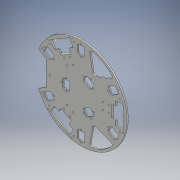
# Autodesk Inventor part: Base
Saved by Autodesk Inventor 2018 (Build 220112000, 112)
## iProperties
Created: 2017-10-12
Part Number: Base
Material: Generic
Document SubType Name: Modeling
Designer: BrisbaneMatt
Density: 1 g/cm^3
Appearance: Default
Author: BrisbaneMatt
Autodesk Inventor part; units mm, degrees
(part 1 of 2)
ref_plane "YZ Plane" through (0, 0, 0) normal (1, 0, 0) x (0, 1, 0)
ref_plane "XZ Plane" through (0, 0, 0) normal (0, 1, 0) x (-1, 0, 0)
ref_plane "XY Plane" through (0, 0, 0) normal (0, 0, 1) x (1, 0, 0)
sketch "Sketch1" plane through (0, 0, 0) normal (0, 1, 0) x (-1, 0, 0)
  circle A0 centre (0, 0) radius 105
  line L0 (0, 0) -> (105, 0) construction
  line L1 (70.1408, 71.4875) -> (26.8396, 96.4875)
  line L2 (70.1408, 71.4875) -> (61.3908, 56.332)
  line L3 (61.3908, 56.332) -> (18.0896, 81.332)
  line L4 (18.0896, 81.332) -> (26.8396, 96.4875)
  line L5 (26.8396, -96.4875) -> (70.1408, -71.4875)
  line L6 (70.1408, -71.4875) -> (61.3908, -56.332)
  line L7 (61.3908, -56.332) -> (18.0896, -81.332)
  line L8 (18.0896, -81.332) -> (26.8396, -96.4875)
  line L9 (0, 0) -> (-105, 0)
  line L10 (-96.9804, -25) -> (-96.9804, 25)
  line L11 (-96.9804, 25) -> (-79.4804, 25)
  line L12 (-79.4804, 25) -> (-79.4804, -25)
  line L13 (-79.4804, -25) -> (-96.9804, -25)
  dimension "d0" = 210
  dimension "d5" = 50
  dimension "d6" = 17.5
  dimension "d8" = 50
  dimension "d9" = 17.5
  dimension "d12" = 50
  dimension "d13" = 17.5
  constraints: 28 end point, 6 perpendicular, 3 horizontal, 1 coincident, 1 horizontal alignment, 1 vertical, 2 other
  measures "d5" distance of L1.start L1.end
  measures "d6" distance of L1.start L2.end
  measures "d8" distance of L5.start L5.end
  measures "d9" distance of L5.end L6.end
  measures "d12" distance of L10.start L10.end
  measures "d13" distance of L10.end L11.end
extrude "Extrusion1" add sketch "Sketch1" along normal blind 3
sketch "Sketch2" plane through (0, 3, 0) normal (0, 1, 0) x (1, 0, 0)
  line L0 (-61.3908, -56.332) -> (-18.0896, -81.332) projected
  line L1 (-39.7402, -68.832) -> (-24.9902, -43.2843)
  line L2 (-32.3652, -56.0582) -> (-35.7652, -61.9471)
  line L3 (-35.7652, -61.9471) -> (-42.6501, -57.9721)
  line L4 (-35.7652, -61.9471) -> (-28.9652, -50.1692)
  line L5 (-28.9652, -50.1692) -> (-35.8501, -46.1942)
  line L6 (-35.8501, -46.1942) -> (-22.0803, -54.1442)
  line L7 (-42.6501, -57.9721) -> (-28.8803, -65.9221)
  circle A0 centre (-42.6501, -57.9721) radius 1.5
  circle A1 centre (-35.8501, -46.1942) radius 1.5
  circle A2 centre (-22.0803, -54.1442) radius 1.5
  circle A3 centre (-28.8803, -65.9221) radius 1.5
  point P0 (0, 0)
  dimension "d17" = 29.5
  dimension "d18" = 6.8
  dimension "d19" = 7.95
  dimension "d20" = 13.6
  dimension "d21" = 7.95
  dimension "d22" = 15.9
  dimension "d23" = 15.9
  dimension "d24" = 3
  dimension "d25" = 3
  dimension "d26" = 3
  dimension "d27" = 3
  constraints: 14 end point, 4 centre point, 4 coincident, 4 point on line, 2 midpoint, 1 perpendicular
  measures "d17" distance of L1.start L1.end
  measures "d18" distance of L2.start L2.end
  measures "d19" distance of L2.end L3.end
  measures "d20" distance of L2.end L4.end
  measures "d21" distance of L4.end L5.end
  measures "d22" distance of L5.end L6.end
  measures "d23" distance of L3.end L7.end
  measures "d24" diameter of A0
  measures "d25" diameter of A1
  measures "d26" diameter of A2
  measures "d27" diameter of A3
extrude "Extrusion2" cut sketch "Sketch2" against normal blind 3
sketch "Sketch3" plane through (0, 3, 0) normal (0, 1, 0) x (1, 0, 0)
  line L0 (-17.4161, -70.8938) -> (-32.5784, -70.8938)
  line L1 (-32.5784, -70.8938) -> (-32.5784, -46.1015)
  line L2 (-32.5784, -46.1015) -> (-17.4161, -46.1015)
  line L3 (-17.4161, -46.1015) -> (-17.4161, -70.8938)
  line L4 (-30.5294, -62.4931) -> (-47.7406, -62.4931)
  line L5 (-47.7406, -62.4931) -> (-47.7406, -39.5448)
  line L6 (-47.7406, -39.5448) -> (-30.5294, -39.5448)
  line L7 (-30.5294, -39.5448) -> (-30.5294, -62.4931)
  point P0 (0, 0)
  constraints: 16 end point, 4 parallel, 2 horizontal, 2 perpendicular
extrude "Extrusion3" add sketch "Sketch3" against normal blind 3
sketch "Sketch4" plane through (0, 3, 0) normal (0, 1, 0) x (1, 0, 0)
  line L0 (-18.0896, -81.332) -> (-61.3908, -56.332) projected
  line L1 (-39.7402, -68.832) -> (-32.812, -72.832)
  line L2 (-32.812, -72.832) -> (-39.7402, -68.832)
  line L3 (-39.7402, -68.832) -> (-35.7402, -61.9038)
  line L4 (-35.7402, -61.9038) -> (-47.4315, -55.1538)
  line L5 (-47.4315, -55.1538) -> (-51.4315, -62.082)
  line L6 (-51.4315, -62.082) -> (-39.7402, -68.832)
  line L7 (-35.7402, -61.9038) -> (-24.0489, -68.6538)
  line L8 (-24.0489, -68.6538) -> (-28.0489, -75.582)
  line L9 (-28.0489, -75.582) -> (-32.812, -72.832)
  line L10 (-61.3908, 56.332) -> (-18.0896, 81.332) projected
  line L11 (-39.7402, 68.832) -> (-51.4315, 62.082)
  line L12 (-51.4315, 62.082) -> (-47.4315, 55.1538)
  line L13 (-47.4315, 55.1538) -> (-24.0489, 68.6538)
  line L14 (-24.0489, 68.6538) -> (-28.0489, 75.582)
  line L15 (-28.0489, 75.582) -> (-39.7402, 68.832)
  line L16 (79.4804, 25) -> (79.4804, -25) projected
  line L17 (79.4804, 0) -> (79.4804, 13.5)
  line L18 (79.4804, 13.5) -> (71.4804, 13.5)
  line L19 (71.4804, 13.5) -> (71.4804, -13.5)
  line L20 (71.4804, -13.5) -> (79.4804, -13.5)
  line L21 (79.4804, -13.5) -> (79.4804, 0)
  point P0 (0, 0)
  dimension "d32" = 8
  dimension "d33" = 8
  dimension "d34" = 13.5
  dimension "d35" = 13.5
  dimension "d36" = 13.5
  dimension "d37" = 8
  dimension "d38" = 27
  dimension "d39" = 13.5
  dimension "d40" = 8
  dimension "d41" = 27
  constraints: 38 end point, 10 perpendicular, 8 point on line, 4 collinear, 3 midpoint
  measures "d32" distance of L1.start L1.end
  measures "d33" distance of L1.start L3.end
  measures "d34" distance of L3.end L4.end
  measures "d35" distance of L3.end L7.end
  measures "d36" distance of L11.start L11.end
  measures "d37" distance of L11.end L12.end
  measures "d38" distance of L12.end L13.end
  measures "d39" distance of L17.start L17.end
  measures "d40" distance of L17.end L18.end
  measures "d41" distance of L18.end L19.end
extrude "Extrusion4" cut sketch "Sketch4" against normal blind 3
sketch "Sketch5" plane through (0, 3, 0) normal (0, 1, 0) x (1, 0, 0)
  line L0 (-47.4315, -55.1538) -> (-24.0489, -68.6538) projected
  line L1 (-35.7402, -61.9038) -> (-4.2402, -7.3442)
  line L2 (-4.2402, -7.3442) -> (-15.9315, -0.5942)
  line L3 (-15.9315, -0.5942) -> (-47.4315, -55.1538)
  line L4 (-4.2402, -7.3442) -> (7.4511, -14.0942)
  line L5 (7.4511, -14.0942) -> (-24.0489, -68.6538)
  line L6 (-24.0489, -68.6538) -> (-35.7402, -61.9038)
  line L7 (-47.4315, 55.1538) -> (-24.0489, 68.6538) projected
  line L8 (-35.7402, 61.9038) -> (-4.2402, 7.3442)
  line L9 (-4.2402, 7.3442) -> (-15.9315, 0.5942)
  line L10 (-47.4315, 55.1538) -> (-51.4315, 62.082) projected
  line L11 (-15.9315, 0.5942) -> (-47.4315, 55.1538)
  line L12 (-47.4315, 55.1538) -> (-24.0489, 68.6538)
  line L13 (-24.0489, 68.6538) -> (7.4511, 14.0942)
  line L14 (7.4511, 14.0942) -> (-4.2402, 7.3442)
  line L15 (71.4804, 13.5) -> (71.4804, -13.5) projected
  line L16 (71.4804, -13.5) -> (8.4804, -13.5)
  line L17 (71.4804, -13.5) -> (134.4804, -13.5) construction
  line L18 (79.4804, 13.5) -> (71.4804, 13.5) projected
  line L19 (71.4804, 13.5) -> (8.4804, 13.5)
  line L20 (71.4804, 13.5) -> (134.4804, 13.5) construction
  line L21 (8.4804, 13.5) -> (8.4804, -13.5)
  line L22 (-35.7402, -61.9038) -> (-47.4315, -55.1538)
  line L23 (0, 0) -> (-30, 0)
  line L24 (-30, 0) -> (-30, -10)
  line L25 (-30, -10) -> (-46, -10)
  line L26 (-46, -10) -> (-46, 10)
  line L27 (-46, 10) -> (-30, 10)
  line L28 (-30, 10) -> (-30, 0)
  line L29 (0, 0) -> (15, 25.9808)
  line L30 (15, 25.9808) -> (6.3397, 30.9808)
  line L31 (6.3397, 30.9808) -> (14.3397, 44.8372)
  line L32 (14.3397, 44.8372) -> (31.6603, 34.8372)
  line L33 (31.6603, 34.8372) -> (23.6603, 20.9808)
  line L34 (23.6603, 20.9808) -> (15, 25.9808)
  line L35 (0, 0) -> (15, -25.9808)
  line L36 (15, -25.9808) -> (6.3397, -30.9808)
  line L37 (6.3397, -30.9808) -> (14.3397, -44.8372)
  line L38 (14.3397, -44.8372) -> (31.6603, -34.8372)
  line L39 (31.6603, -34.8372) -> (23.6603, -20.9808)
  line L40 (23.6603, -20.9808) -> (15, -25.9808)
  dimension "d45" = 63
  dimension "d46" = 13.5
  dimension "d47" = 13.5
  dimension "d49" = 63
  dimension "d50" = 13.5
  dimension "d51" = 63
  dimension "d52" = 180
  dimension "d53" = 63
  dimension "d54" = 180
  dimension "d55" = 30
  dimension "d56" = 10
  dimension "d57" = 16
  dimension "d58" = 20
  dimension "d59" = 30
  dimension "d60" = 10
  dimension "d61" = 16
  dimension "d62" = 20
  dimension "d63" = 30
  dimension "d64" = 10
  dimension "d65" = 16
  dimension "d66" = 20
  constraints: 72 end point, 20 perpendicular, 5 point on line, 4 collinear, 4 horizontal, 2 midpoint
  measures "d45" distance of L1.start L1.end
  measures "d46" distance of L1.end L2.end
  measures "d47" distance of L1.end L4.end
  measures "d49" distance of L8.start L8.end
  measures "d50" distance of L8.end L9.end
  measures "d51" distance of L15.end L16.end
  measures "d52" angle of L16 L17
  measures "d53" distance of L15.start L19.end
  measures "d54" angle of L19 L20
  measures "d55" distance of L23.start L23.end
  measures "d56" distance of L23.end L24.end
  measures "d57" distance of L24.end L25.end
  measures "d58" distance of L25.end L26.end
  measures "d59" distance of L23.start L29.end
  measures "d60" distance of L29.end L30.end
  measures "d61" distance of L30.end L31.end
  measures "d62" distance of L31.end L32.end
  measures "d63" distance of L23.start L35.end
  measures "d64" distance of L35.end L36.end
  measures "d65" distance of L36.end L37.end
  measures "d66" distance of L37.end L38.end
extrude "Extrusion5" cut sketch "Sketch5" against normal blind 3 contours L24 L25 L26 L27 L28 | L30 L31 L32 L33 L34 | L40 L39 L38 L37 L36
sketch "Sketch6" plane through (0, 3, 0) normal (0, 1, 0) x (1, 0, 0)
  line L0 (0, 0) -> (-77.9423, -45)
  line L1 (0, 0) -> (90, 0) construction
  line L2 (-77.9423, -45) -> (-82.2724, -47.5)
  line L3 (-82.2724, -47.5) -> (-87.2724, -38.8397)
  line L4 (-87.2724, -38.8397) -> (-73.416, -30.8397)
  line L5 (-73.416, -30.8397) -> (-63.416, -48.1603)
  line L6 (-63.416, -48.1603) -> (-77.2724, -56.1603)
  line L7 (-77.2724, -56.1603) -> (-82.2724, -47.5)
  line L8 (0, 0) -> (90, 0) construction
  line L9 (0, 0) -> (0, 95)
  line L10 (0, 0) -> (-82.2724, 47.5)
  line L11 (0, 0) -> (95, 0) construction
  line L12 (-82.2724, 47.5) -> (-77.2724, 56.1603)
  line L13 (-77.2724, 56.1603) -> (-63.416, 48.1603)
  line L14 (-63.416, 48.1603) -> (-73.416, 30.8397)
  line L15 (-73.416, 30.8397) -> (-87.2724, 38.8397)
  line L16 (-87.2724, 38.8397) -> (-82.2724, 47.5)
  line L17 (0, 95) -> (-10, 95)
  line L18 (-10, 95) -> (-10, 79)
  line L19 (-10, 79) -> (10, 79)
  line L20 (10, 79) -> (10, 95)
  line L21 (10, 95) -> (0, 95)
  line L22 (0, 0) -> (82.2724, 47.5)
  line L23 (82.2724, 47.5) -> (77.2724, 56.1603)
  line L24 (77.2724, 56.1603) -> (63.416, 48.1603)
  line L25 (63.416, 48.1603) -> (73.416, 30.8397)
  line L26 (73.416, 30.8397) -> (87.2724, 38.8397)
  line L27 (87.2724, 38.8397) -> (82.2724, 47.5)
  line L28 (0, 0) -> (82.2724, -47.5)
  line L29 (82.2724, -47.5) -> (77.2724, -56.1603)
  line L30 (77.2724, -56.1603) -> (63.416, -48.1603)
  line L31 (63.416, -48.1603) -> (73.416, -30.8397)
  line L32 (73.416, -30.8397) -> (87.2724, -38.8397)
  line L33 (82.2724, -47.5) -> (87.2724, -38.8397)
  line L34 (0, 0) -> (0, -95)
  line L35 (0, -95) -> (-10, -95)
  line L36 (-10, -95) -> (-10, -79)
  line L37 (-10, -79) -> (10, -79)
  line L38 (10, -79) -> (10, -95)
  line L39 (0, -95) -> (10, -95)
  dimension "d69" = 90
  dimension "d70" = 150
  dimension "d71" = 5
  dimension "d72" = 10
  dimension "d73" = 16
  dimension "d74" = 20
  dimension "d80" = 95
  dimension "d81" = 95
  dimension "d82" = 150
  dimension "d83" = 10
  dimension "d84" = 10
  dimension "d85" = 16
  dimension "d86" = 20
  dimension "d87" = 95
  dimension "d88" = 10
  dimension "d89" = 16
  dimension "d90" = 20
  dimension "d91" = 16
  constraints: 80 end point, 26 perpendicular, 15 point on line, 4 horizontal, 2 equal length, 1 vertical
  measures "d69" distance of L0.start L0.end
  measures "d70" angle of L0 L1
  measures "d71" distance of L0.end L2.end
  measures "d72" distance of L2.end L3.end
  measures "d73" distance of L3.end L4.end
  measures "d74" distance of L4.end L5.end
  measures "d80" distance of L0.start L9.end
  measures "d81" distance of L0.start L10.end
  measures "d82" angle of L11 L10
  measures "d83" distance of L10.end L12.end
  measures "d84" distance of L9.end L17.end
  measures "d85" distance of L17.end L18.end
  measures "d86" distance of L18.end L19.end
  measures "d87" distance of L0.start L22.end
  measures "d88" distance of L22.end L23.end
  measures "d89" distance of L23.end L24.end
  measures "d90" distance of L24.end L25.end
  measures "d91" distance of L35.end L36.end
extrude "Extrusion6" cut sketch "Sketch6" against normal blind 3
sketch "Sketch7" plane through (0, 3, 0) normal (0, 1, 0) x (1, 0, 0)
  line L0 (-47.4315, 55.1538) -> (-24.0489, 68.6538) projected
  line L1 (-35.7402, 61.9038) -> (-20.9902, 36.3561)
  line L2 (-28.3652, 49.13) -> (-31.7652, 55.0189)
  line L3 (-31.7652, 55.0189) -> (-38.6501, 51.0439)
  line L4 (-38.6501, 51.0439) -> (-24.8803, 58.9939)
  line L5 (-28.3652, 49.13) -> (-24.9652, 43.241)
  line L6 (-24.9652, 43.241) -> (-31.8501, 39.266)
  line L7 (-31.8501, 39.266) -> (-18.0803, 47.216)
  circle A0 centre (-31.8501, 39.266) radius 1.5
  circle A1 centre (-38.6501, 51.0439) radius 1.5
  circle A2 centre (-24.8803, 58.9939) radius 1.5
  circle A3 centre (-18.0803, 47.216) radius 1.5
  line L8 (71.4804, 13.5) -> (71.4804, -13.5) projected
  line L9 (71.4804, 0) -> (41.9804, 0)
  line L10 (41.9804, 0) -> (56.7304, 0)
  line L11 (56.7304, 0) -> (63.5304, 0)
  line L12 (63.5304, 0) -> (49.9304, 0)
  line L13 (49.9304, 0) -> (49.9304, 7.95)
  line L14 (49.9304, 7.95) -> (49.9304, -7.95)
  line L15 (63.5304, 0) -> (63.5304, 7.95)
  line L16 (63.5304, 7.95) -> (63.5304, -7.95)
  circle A4 centre (49.9304, -7.95) radius 1.5
  circle A5 centre (49.9304, 7.95) radius 1.5
  circle A6 centre (63.5304, 7.95) radius 1.5
  circle A7 centre (63.5304, -7.95) radius 1.5
  line L17 (-24.0489, -68.6538) -> (-47.4315, -55.1538) projected
  line L18 (-35.7402, -61.9038) -> (-10.1924, -76.6538)
  line L19 (-10.1924, -76.6538) -> (-35.7402, -61.9038)
  line L20 (-35.7402, -61.9038) -> (-20.9902, -36.3561)
  line L21 (-28.3652, -49.13) -> (-24.9652, -43.241)
  line L22 (-24.9652, -43.241) -> (-31.7652, -55.0189)
  line L23 (-31.7652, -55.0189) -> (-38.6501, -51.0439)
  line L24 (-38.6501, -51.0439) -> (-24.8803, -58.9939)
  line L25 (-24.9652, -43.241) -> (-31.8501, -39.266)
  line L26 (-24.9652, -43.241) -> (-17.0152, -43.241) construction
  line L27 (-31.8501, -39.266) -> (-18.0803, -47.216)
  circle A8 centre (-38.6501, -51.0439) radius 1.5
  circle A9 centre (-31.8501, -39.266) radius 1.5
  circle A10 centre (-18.0803, -47.216) radius 1.5
  circle A11 centre (-24.8803, -58.9939) radius 1.5
  point P0 (0, 0)
  dimension "d95" = 29.5
  dimension "d96" = 6.8
  dimension "d97" = 7.95
  dimension "d98" = 15.9
  dimension "d99" = 6.8
  dimension "d100" = 7.95
  dimension "d101" = 15.9
  dimension "d102" = 3
  dimension "d103" = 3
  dimension "d104" = 3
  dimension "d105" = 3
  dimension "d106" = 29.5
  dimension "d107" = 6.8
  dimension "d108" = 13.6
  dimension "d109" = 7.95
  dimension "d110" = 15.9
  dimension "d111" = 7.95
  dimension "d112" = 15.9
  dimension "d113" = 3
  dimension "d114" = 3
  dimension "d115" = 3
  dimension "d116" = 3
  dimension "d117" = 29.5
  dimension "d118" = 29.5
  dimension "d119" = 6.8
  dimension "d120" = 13.6
  dimension "d121" = 7.95
  dimension "d122" = 15.9
  dimension "d123" = 7.95
  dimension "d124" = 150
  dimension "d125" = 15.9
  dimension "d126" = 3
  dimension "d127" = 3
  dimension "d128" = 3
  dimension "d129" = 3
  constraints: 50 end point, 12 centre point, 12 coincident, 12 point on line, 6 midpoint, 5 perpendicular, 2 collinear, 2 horizontal, 1 equal length, 1 vertical
  measures "d95" distance of L1.start L1.end
  measures "d96" distance of L2.start L2.end
  measures "d97" distance of L2.end L3.end
  measures "d98" distance of L3.end L4.end
  measures "d99" distance of L2.start L5.end
  measures "d100" distance of L5.end L6.end
  measures "d101" distance of L6.end L7.end
  measures "d102" diameter of A0
  measures "d103" diameter of A1
  measures "d104" diameter of A2
  measures "d105" diameter of A3
  measures "d106" distance of L9.start L9.end
  measures "d107" distance of L10.end L11.end
  measures "d108" distance of L11.end L12.end
  measures "d109" distance of L12.end L13.end
  measures "d110" distance of L13.end L14.end
  measures "d111" distance of L11.end L15.end
  measures "d112" distance of L15.end L16.end
  measures "d113" diameter of A4
  measures "d114" diameter of A5
  measures "d115" diameter of A6
  measures "d116" diameter of A7
  measures "d117" distance of L18.start L18.end
  measures "d118" distance of L18.start L20.end
  measures "d119" distance of L21.start L21.end
  measures "d120" distance of L21.end L22.end
  measures "d121" distance of L22.end L23.end
  measures "d122" distance of L23.end L24.end
  measures "d123" distance of L21.end L25.end
  measures "d124" angle of L26 L25
  measures "d125" distance of L25.end L27.end
  measures "d126" diameter of A8
  measures "d127" diameter of A9
  measures "d128" diameter of A10
  measures "d129" diameter of A11
extrude "Extrusion7" cut sketch "Sketch7" against normal blind 3
sketch "Sketch8" plane through (0, 3, 0) normal (0, 1, 0) x (1, 0, 0)
  line L0 (-73.416, -30.8397) -> (-87.2724, -38.8397) projected
  line L1 (-80.3442, -34.8397) -> (-84.6743, -37.3397)
  line L2 (-84.6743, -37.3397) -> (-87.1743, -33.0096)
  line L3 (-87.1743, -33.0096) -> (-97.5, -38.9711)
  circle A0 centre (0, 0) radius 105 projected
  line L4 (-73.416, 30.8397) -> (-87.2724, 38.8397) projected
  line L5 (-80.3442, 34.8397) -> (-84.6743, 37.3397)
  line L6 (-84.6743, 37.3397) -> (-87.1743, 33.0096)
  line L7 (-87.1743, 33.0096) -> (-97.5, 38.9711)
  line L8 (-105, 0) -> (-80, 0)
  line L9 (-80, 0) -> (-80, -28.8675)
  line L10 (-80, -28.8675) -> (-87.1743, -33.0096)
  line L11 (-80, 0) -> (-80, 28.8675)
  line L12 (-80, 28.8675) -> (-87.1743, 33.0096)
  arc A1 (-97.5, 38.9711) -> (-97.5, -38.9711) centre (0, 0) ccw
  dimension "d132" = 5
  dimension "d133" = 5
  dimension "d134" = 5
  dimension "d135" = 5
  dimension "d136" = 25
  constraints: 22 end point, 6 perpendicular, 5 point on circle, 4 point on line, 2 midpoint, 1 centre point, 1 horizontal
  measures "d132" distance of L1.start L1.end
  measures "d133" distance of L1.end L2.end
  measures "d134" distance of L5.start L5.end
  measures "d135" distance of L5.end L6.end
  measures "d136" distance of L8.start L8.end
extrude "Extrusion8" cut sketch "Sketch8" against normal blind 3 contours L3 A0 L8 L9 L10
sketch "Sketch9" plane through (0, 3, 0) normal (0, 1, 0) x (1, 0, 0)
  line L0 (-80, -28.8675) -> (-80, 0) projected
  line L1 (-80, 0) -> (-80, 26.0144)
  line L2 (-73.416, 30.8397) -> (-87.2724, 38.8397) projected
  line L3 (-80.3442, 34.8397) -> (-84.6743, 37.3397)
  line L4 (-84.6743, 37.3397) -> (-80.3442, 34.8397)
  line L5 (-80.3442, 34.8397) -> (-82.8442, 30.5096)
  line L6 (-82.8442, 30.5096) -> (-80, 28.8675)
  line L7 (-80, 28.8675) -> (-80, 26.0144)
  line L8 (-82.8442, 30.5096) -> (-97.5, 38.9711)
  arc A0 (-97.5, -38.9711) -> (-105, 0) centre (0, 0) ccw projected
  line L9 (-105, 0) -> (-80, 0) projected
  line L10 (-80, 0) -> (-105, 0)
  arc A1 (-97.5, 38.9711) -> (-105, 0) centre (0, 0) ccw
  dimension "d139" = 5
  dimension "d140" = 5
  constraints: 16 end point, 3 point on circle, 2 collinear, 2 perpendicular, 2 point on line, 2 vertical, 1 centre point, 1 concentric, 1 midpoint
  measures "d139" distance of L3.start L3.end
  measures "d140" distance of L3.start L5.end
extrude "Extrusion9" cut sketch "Sketch9" against normal blind 3
sketch "Sketch10" plane through (0, 3, 0) normal (0, 1, 0) x (1, 0, 0)
  line L0 (-70.1408, 71.4875) -> (-61.3908, 56.332) projected
  circle A0 centre (0, 0) radius 100.1509
  circle A1 centre (0, 0) radius 102.651
  line L1 (0, 0) -> (-65.7658, 63.9098)
  line L2 (-65.7658, 63.9098) -> (-73.6166, 71.539)
  line L3 (0, 0) -> (-22.4646, 88.9098)
  line L4 (-26.8396, 96.4875) -> (-18.0896, 81.332) projected
  line L5 (-25.1463, 99.5233) -> (-22.4646, 88.9098)
  line L6 (0, 0) -> (88.2304, 25)
  line L7 (96.9804, 25) -> (79.4804, 25) projected
  line L8 (88.2304, 25) -> (98.7629, 27.9844)
  line L9 (0, 0) -> (88.2304, -25)
  line L10 (79.4804, -25) -> (96.9804, -25) projected
  line L11 (88.2304, -25) -> (98.7629, -27.9844)
  line L12 (0, 0) -> (-22.4646, -88.9098)
  line L13 (-18.0896, -81.332) -> (-26.8396, -96.4875) projected
  line L14 (-22.4646, -88.9098) -> (-21.4622, -84.9428)
  line L15 (-21.4622, -84.9428) -> (-23.9119, -94.6381)
  line L16 (-23.9119, -94.6381) -> (-25.1463, -99.5233)
  line L17 (0, 0) -> (-65.7658, -63.9098)
  line L18 (-70.1408, -71.4875) -> (-61.3908, -56.332) projected
  line L19 (-65.7658, -63.9098) -> (-62.2668, -60.5095)
  line L20 (-62.2668, -60.5095) -> (-70.8726, -68.8724)
  line L21 (-70.8726, -68.8724) -> (-73.6166, -71.539)
  dimension "d144" = 205.302
  dimension "d145" = 10
  dimension "d146" = 12
  constraints: 32 end point, 10 point on line, 7 point on circle, 6 midpoint, 2 centre point, 2 coincident, 1 collinear
  measures "d144" diameter of A1
  measures "d145" distance of L14.end L15.end
  measures "d146" distance of L19.end L20.end
extrude "Extrusion10" add sketch "Sketch10" along normal blind 3 contours A0 L2 A1 L5 | L0 L2 A0 | A0 L5 L4 | L12 L13 A0 L18 L17 | L21 L20 L18 A0 | A0 L16 A1 L21 | L8 A0 L7 | L10 A0 L11 | L8 A1 L11 A0 | L15 L16 A0 L13
sketch "Sketch11" plane through (0, 6, 0) normal (0, 1, 0) x (1, 0, 0)
  line L0 (-26.8396, -96.4875) -> (-18.0896, -81.332) projected
  line L1 (-26.8396, -96.4875) -> (-22.4646, -88.9098)
  line L2 (-70.1408, -71.4875) -> (-26.8396, -96.4875) projected
  circle A0 centre (0, 0) radius 100.1509
  line L3 (-22.4646, -88.9098) -> (-24.5338, -97.0994)
  line L4 (-22.4646, -88.9098) -> (-25.1463, -99.5233) projected
  line L5 (-59.2437, -57.5717) -> (-65.7658, -63.9098) projected
  line L6 (-61.3908, -56.332) -> (-70.1408, -71.4875) projected
  line L7 (-65.7658, -63.9098) -> (-70.1408, -71.4875)
  line L8 (-65.7658, -63.9098) -> (-71.8236, -69.7966)
  constraints: 8 end point, 3 point on circle, 2 point on line, 1 centre point, 1 coincident, 1 collinear, 1 midpoint
extrude "Extrusion11" cut sketch "Sketch11" against normal blind 3 contours L2 L6 L8 A0 L3 L0
sketch "Sketch12" plane through (0, 6, 0) normal (0, 1, 0) x (1, 0, 0)
  arc A0 (96.9804, -25) -> (96.9804, 25) centre (0, 0) ccw projected
  circle A1 centre (0, 0) radius 100.1509
  constraints: 1 coincident, 3 other
extrude "Extrusion12" cut sketch "Sketch12" against normal blind 3
sketch "Sketch13" plane through (0, 6, 0) normal (0, 1, 0) x (1, 0, 0)
  line L0 (98.7629, -27.9844) -> (96.3574, -27.3028) projected
  line L1 (96.3574, -27.3028) -> (98.7629, -27.9844)
  line L2 (96.3574, 27.3028) -> (98.7629, 27.9844) projected
  line L3 (96.3574, 27.3028) -> (98.7629, 27.9844)
  arc A0 (98.7629, -27.9844) -> (98.7629, 27.9844) centre (0, 0) ccw projected
  arc A1 (96.3574, -27.3028) -> (96.9804, -25) centre (0, 0) ccw projected
  arc A2 (96.9804, -25) -> (96.3574, 27.3028) centre (0, 0) ccw
  arc A3 (96.9804, -25) -> (96.9804, 25) centre (0, 0) ccw projected
  arc A4 (96.3574, -27.3028) -> (96.9804, -25) centre (0, 0) ccw
  arc A5 (98.7629, -27.9844) -> (98.7629, 27.9844) centre (0, 0) ccw
  constraints: 6 point on circle, 4 end point, 3 centre point, 2 collinear, 1 concentric
extrude "Extrusion13" add sketch "Sketch13" along normal blind 27
sketch "Sketch14" plane through (0, 6, 0) normal (0, 1, 0) x (1, 0, 0)
  line L0 (-73.6166, -71.539) -> (-71.8236, -69.7966) projected
  line L1 (-24.5338, -97.0994) -> (-25.1463, -99.5233) projected
  arc A0 (-73.6166, -71.539) -> (-25.1463, -99.5233) centre (0, 0) ccw
  arc A1 (-71.8236, -69.7966) -> (-70.1408, -71.4875) centre (0, 0) ccw projected
  arc A2 (-26.8396, -96.4875) -> (-24.5338, -97.0994) centre (0, 0) ccw projected
  arc A3 (-70.1408, -71.4875) -> (-26.8396, -96.4875) centre (0, 0) ccw
  constraints: 4 point on circle, 2 centre point
extrude "Extrusion14" add sketch "Sketch14" along normal blind 27
sketch "Sketch15" plane through (0, 6, 0) normal (0, 1, 0) x (1, 0, 0)
  arc A0 (-25.1463, 99.5233) -> (-73.6166, 71.539) centre (0, 0) ccw projected
  arc A1 (-73.6166, 71.539) -> (-25.1463, 99.5233) centre (0, 0) ccw
  line L0 (-25.1463, 99.5233) -> (-24.5338, 97.0994) projected
  arc A2 (-70.1408, 71.4875) -> (-71.8236, 69.7966) centre (0, 0) ccw projected
  arc A3 (-24.5338, 97.0994) -> (-70.1408, 71.4875) centre (0, 0) ccw
  line L1 (-71.8236, 69.7966) -> (-73.6166, 71.539) projected
  line L2 (-71.8236, 69.7966) -> (-73.6166, 71.539)
  constraints: 4 point on circle, 2 centre point, 2 end point, 1 collinear
extrude "Extrusion15" add sketch "Sketch15" along normal blind 27 contours L0 A3 A2 L1 A0
fillet "Fillet1" radius 2 6 edges at (-28.0489, 1.5, -75.582) (-51.4315, 1.5, -62.082) (79.4804, 1.5, -13.5) (79.4804, 1.5, 13.5) (-28.0489, 1.5, 75.582) (-51.4315, 1.5, 62.082)
fillet "Fillet2" radius 2 4 edges at (73.416, 1.5, 30.8397) (87.2724, 1.5, 38.8397) (63.416, 1.5, 48.1603) (77.2724, 1.5, 56.1603)
fillet "Fillet3" radius 2 4 edges at (23.6603, 1.5, 20.9808) (6.3397, 1.5, 30.9808) (14.3397, 1.5, 44.8372) (31.6603, 1.5, 34.8372)
fillet "Fillet4" radius 2 4 edges at (10, 1.5, 79) (-10, 1.5, 79) (-10, 1.5, 95) (10, 1.5, 95)
fillet "Fillet5" radius 2 4 edges at (-30, 1.5, -10) (-46, 1.5, -10) (-46, 1.5, 10) (-30, 1.5, 10)
fillet "Fillet6" radius 2 4 edges at (-73.416, 1.5, 30.8397) (-87.2724, 1.5, 38.8397) (-77.2724, 1.5, 56.1603) (-63.416, 1.5, 48.1603)
fillet "Fillet7" radius 2 4 edges at (-63.416, 1.5, -48.1603) (-73.416, 1.5, -30.8397) (-87.2724, 1.5, -38.8397) (-77.2724, 1.5, -56.1603)
fillet "Fillet8" radius 2 4 edges at (6.3397, 1.5, -30.9808) (31.6603, 1.5, -34.8372) (23.6603, 1.5, -20.9808) (14.3397, 1.5, -44.8372)
fillet "Fillet9" radius 2 4 edges at (77.2724, 1.5, -56.1603) (63.416, 1.5, -48.1603) (73.416, 1.5, -30.8397) (87.2724, 1.5, -38.8397)
fillet "Fillet10" radius 2 4 edges at (-10, 1.5, -95) (10, 1.5, -95) (10, 1.5, -79) (-10, 1.5, -79)
sketch "Sketch16" plane through (0, 3, 0) normal (0, 1, 0) x (1, 0, 0)
  line L0 (-80, 28.8675) -> (-80, -28.8675) projected
  line L1 (-80, -26.5025) -> (-80, -23.5025)
  line L2 (-80, -23.5025) -> (-80, -26.5025)
  line L3 (-80, -26.5025) -> (-77, -26.5025)
  line L4 (-80, -28.8675) -> (-97.5, -38.9711) projected
  line L5 (-86.295, -32.5019) -> (-83.6969, -31.0019)
  line L6 (-83.6969, -31.0019) -> (-82.1969, -33.6)
  line L7 (-82.1969, -33.6) -> (-77, -30.5996)
  line L8 (-77, -30.5996) -> (-77, -26.5025)
  line L9 (-82.1969, -33.6) -> (-96.3369, -41.7637)
  arc A0 (-97.5, -38.9711) -> (-97.5, 38.9711) centre (0, 0) ccw projected
  line L10 (-97.5, 38.9711) -> (-80, 28.8675) projected
  line L11 (-82.9469, 30.5689) -> (-80.3488, 29.0689)
  line L12 (-80.3488, 29.0689) -> (-82.9469, 30.5689)
  line L13 (-82.9469, 30.5689) -> (-81.4469, 33.167)
  line L14 (-77, -26.5025) -> (-77, 30.5996)
  line L15 (-77, 30.5996) -> (-81.4469, 33.167)
  line L16 (-81.4469, 33.167) -> (-96.3369, 41.7637)
  dimension "d169" = 3
  dimension "d170" = 3
  dimension "d171" = 3
  dimension "d172" = 3
  dimension "d173" = 3
  dimension "d174" = 3
  constraints: 28 end point, 8 point on line, 4 perpendicular, 2 collinear, 2 point on circle, 2 vertical
  measures "d169" distance of L1.start L1.end
  measures "d170" distance of L1.start L3.end
  measures "d171" distance of L5.start L5.end
  measures "d172" distance of L5.end L6.end
  measures "d173" distance of L11.start L11.end
  measures "d174" distance of L11.start L13.end
extrude "Extrusion16" add sketch "Sketch16" along normal blind 30 contours L10 L13 L15 L14 L3 L0 | L3 L8 L7 L6 L4 L0 | L10 A0 L16 L13 | L6 L9 A0 L4
sketch "Sketch17" plane through (-80, 0, -28.8675) normal (-1, 0, 0) x (0, 0, 1)
  line L0 (4.8327, 31.418) -> (62.2102, 31.418) construction
  line L1 (62.2102, 31.418) -> (62.2102, 22.5452) construction
  line L2 (62.2102, 22.5452) -> (4.8327, 22.5452) construction
  line L3 (4.8327, 22.5452) -> (4.8327, 31.418) construction
  line L4 (46.696, 31.418) -> (46.696, 22.5452)
  line L5 (46.696, 26.5678) -> (56.1703, 26.5678)
  line L6 (56.1703, 33) -> (56.1703, 3) projected
  line L7 (4.8327, 26.3472) -> (0, 26.3472)
  line L8 (0, 0) -> (0, 33) projected
  line L9 (7.9005, 28.161) -> (7.4752, 28.161)
  line L10 (7.4752, 28.161) -> (7.4752, 30.9175)
  line L11 (7.4752, 30.9175) -> (6.6402, 29.0427)
  line L12 (6.6402, 29.0427) -> (6.3809, 29.0427)
  line L13 (6.3809, 29.0427) -> (5.5536, 30.9175)
  line L14 (5.5536, 30.9175) -> (5.5536, 28.161)
  line L15 (5.5536, 28.161) -> (5.1569, 28.161)
  line L16 (5.1569, 28.161) -> (5.1569, 31.361)
  line L17 (5.1569, 31.361) -> (5.7378, 31.361)
  line L18 (5.7378, 31.361) -> (6.5365, 29.5795)
  line L19 (6.5365, 29.5795) -> (7.3092, 31.361)
  line L20 (7.3092, 31.361) -> (7.9005, 31.361)
  line L21 (7.9005, 31.361) -> (7.9005, 28.161)
  line L22 (8.2039, 28.161) -> (9.2827, 31.361)
  line L23 (9.2827, 31.361) -> (9.8065, 31.361)
  line L24 (9.8065, 31.361) -> (10.8852, 28.161)
  line L25 (10.8852, 28.161) -> (10.4366, 28.161)
  line L26 (10.4366, 28.161) -> (10.1462, 29.0556)
  line L27 (10.1462, 29.0556) -> (8.9248, 29.0556)
  line L28 (8.9248, 29.0556) -> (8.6344, 28.161)
  line L29 (8.6344, 28.161) -> (8.2039, 28.161)
  line L30 (10.0295, 29.4187) -> (9.5342, 30.9253)
  line L31 (9.5342, 30.9253) -> (9.0415, 29.4187)
  line L32 (9.0415, 29.4187) -> (10.0295, 29.4187)
  spline S0 degree 2 poles (13.2113, 30.3963) (13.2113, 30.1889) (13.0635, 29.8154) (12.9313, 29.6858) knots 0 0 0 1 2 2 2
  spline S1 degree 2 poles (12.9313, 29.6858) (12.7653, 29.5224) (12.3167, 29.3539) (11.9744, 29.3539) knots 0 0 0 1 2 2 2
  line L33 (11.9744, 29.3539) -> (11.6139, 29.3539)
  line L34 (11.6139, 29.3539) -> (11.6139, 28.161)
  line L35 (11.6139, 28.161) -> (11.1886, 28.161)
  line L36 (11.1886, 28.161) -> (11.1886, 31.361)
  line L37 (11.1886, 31.361) -> (11.9925, 31.361)
  spline S2 degree 2 poles (11.9925, 31.361) (12.2778, 31.361) (12.6771, 31.2676) (12.8301, 31.1613) knots 0 0 0 1 2 2 2
  spline S3 degree 2 poles (12.8301, 31.1613) (13.0091, 31.0394) (13.2113, 30.6634) (13.2113, 30.3963) knots 0 0 0 1 2 2 2
  spline S4 degree 2 poles (12.7679, 30.3833) (12.7679, 30.5493) (12.6538, 30.7931) (12.5371, 30.8709) knots 0 0 0 1 2 2 2
  spline S5 degree 2 poles (12.5371, 30.8709) (12.436, 30.9383) (12.1663, 30.9927) (11.9666, 30.9927) knots 0 0 0 1 2 2 2
  line L38 (11.9666, 30.9927) -> (11.6139, 30.9927)
  line L39 (11.6139, 30.9927) -> (11.6139, 29.7169)
  line L40 (11.6139, 29.7169) -> (11.9044, 29.7169)
  spline S6 degree 2 poles (11.9044, 29.7169) (12.1637, 29.7169) (12.4827, 29.7999) (12.5864, 29.9088) knots 0 0 0 1 2 2 2
  spline S7 degree 2 poles (12.5864, 29.9088) (12.6823, 30.0047) (12.7679, 30.2303) (12.7679, 30.3833) knots 0 0 0 1 2 2 2
  line L41 (15.47, 28.161) -> (13.6159, 28.161)
  line L42 (13.6159, 28.161) -> (13.6159, 31.361)
  line L43 (13.6159, 31.361) -> (14.0412, 31.361)
  line L44 (14.0412, 31.361) -> (14.0412, 28.5396)
  line L45 (14.0412, 28.5396) -> (15.47, 28.5396)
  line L46 (15.47, 28.5396) -> (15.47, 28.161)
  line L47 (15.8045, 28.161) -> (15.8045, 31.361)
  line L48 (15.8045, 31.361) -> (17.8065, 31.361)
  line L49 (17.8065, 31.361) -> (17.8065, 30.9824)
  line L50 (17.8065, 30.9824) -> (16.2298, 30.9824)
  line L51 (16.2298, 30.9824) -> (16.2298, 30.1059)
  line L52 (16.2298, 30.1059) -> (17.7002, 30.1059)
  line L53 (17.7002, 30.1059) -> (17.7002, 29.7273)
  line L54 (17.7002, 29.7273) -> (16.2298, 29.7273)
  line L55 (16.2298, 29.7273) -> (16.2298, 28.5396)
  line L56 (16.2298, 28.5396) -> (17.8065, 28.5396)
  line L57 (17.8065, 28.5396) -> (17.8065, 28.161)
  line L58 (17.8065, 28.161) -> (15.8045, 28.161)
  spline S8 degree 2 poles (20.4438, 29.1438) (20.4438, 28.9052) (20.2622, 28.5396) (20.1118, 28.4203) knots 0 0 0 1 2 2 2
  spline S9 degree 2 poles (20.1118, 28.4203) (19.9303, 28.2803) (19.518, 28.161) (19.1912, 28.161) knots 0 0 0 1 2 2 2
  line L59 (19.1912, 28.161) -> (18.2732, 28.161)
  line L60 (18.2732, 28.161) -> (18.2732, 31.361)
  line L61 (18.2732, 31.361) -> (19.1212, 31.361)
  spline S10 degree 2 poles (19.1212, 31.361) (19.4635, 31.361) (19.8058, 31.3169) (19.9614, 31.2313) knots 0 0 0 1 2 2 2
  spline S11 degree 2 poles (19.9614, 31.2313) (20.1352, 31.1406) (20.2933, 30.8423) (20.2933, 30.6401) knots 0 0 0 1 2 2 2
  spline S12 degree 2 poles (20.2933, 30.6401) (20.2933, 30.4145) (20.0548, 30.0566) (19.8447, 29.9555) knots 0 0 0 1 2 2 2
  line L62 (19.8447, 29.9555) -> (19.8447, 29.9399)
  spline S13 degree 2 poles (19.8447, 29.9399) (20.13, 29.8621) (20.4438, 29.4498) (20.4438, 29.1438) knots 0 0 0 1 2 2 2
  spline S14 degree 2 poles (20.0003, 29.1256) (20.0003, 29.3072) (19.8966, 29.5406) (19.741, 29.6235) knots 0 0 0 1 2 2 2
  spline S15 degree 2 poles (19.741, 29.6235) (19.6399, 29.6754) (19.4013, 29.7065) (19.1809, 29.7065) knots 0 0 0 1 2 2 2
  line L63 (19.1809, 29.7065) -> (18.6985, 29.7065)
  line L64 (18.6985, 29.7065) -> (18.6985, 28.524)
  line L65 (18.6985, 28.524) -> (19.0434, 28.524)
  spline S16 degree 2 poles (19.0434, 28.524) (19.3235, 28.524) (19.645, 28.5759) (19.7695, 28.6589) knots 0 0 0 1 2 2 2
  spline S17 degree 2 poles (19.7695, 28.6589) (19.8888, 28.7445) (20.0003, 28.9571) (20.0003, 29.1256) knots 0 0 0 1 2 2 2
  spline S18 degree 2 poles (19.8499, 30.5804) (19.8499, 30.6945) (19.7721, 30.8657) (19.6865, 30.915) knots 0 0 0 1 2 2 2
  spline S19 degree 2 poles (19.6865, 30.915) (19.5828, 30.972) (19.3313, 30.9979) (19.1057, 30.9979) knots 0 0 0 1 2 2 2
  line L66 (19.1057, 30.9979) -> (18.6985, 30.9979)
  line L67 (18.6985, 30.9979) -> (18.6985, 30.0618)
  line L68 (18.6985, 30.0618) -> (19.1809, 30.0618)
  spline S20 degree 2 poles (19.1809, 30.0618) (19.3805, 30.0618) (19.5698, 30.1033) (19.671, 30.1681) knots 0 0 0 1 2 2 2
  spline S21 degree 2 poles (19.671, 30.1681) (19.7695, 30.2303) (19.8499, 30.43) (19.8499, 30.5804) knots 0 0 0 1 2 2 2
  line L69 (20.5215, 28.161) -> (21.6003, 31.361)
  line L70 (21.6003, 31.361) -> (22.1241, 31.361)
  line L71 (22.1241, 31.361) -> (23.2029, 28.161)
  line L72 (23.2029, 28.161) -> (22.7543, 28.161)
  line L73 (22.7543, 28.161) -> (22.4638, 29.0556)
  line L74 (22.4638, 29.0556) -> (21.2425, 29.0556)
  line L75 (21.2425, 29.0556) -> (20.952, 28.161)
  line L76 (20.952, 28.161) -> (20.5215, 28.161)
  line L77 (22.3472, 29.4187) -> (21.8519, 30.9253)
  line L78 (21.8519, 30.9253) -> (21.3591, 29.4187)
  line L79 (21.3591, 29.4187) -> (22.3472, 29.4187)
  line L80 (25.9828, 28.161) -> (25.4305, 28.161)
  line L81 (25.4305, 28.161) -> (24.4191, 29.4342)
  line L82 (24.4191, 29.4342) -> (23.9316, 29.4342)
  line L83 (23.9316, 29.4342) -> (23.9316, 28.161)
  line L84 (23.9316, 28.161) -> (23.5063, 28.161)
  line L85 (23.5063, 28.161) -> (23.5063, 31.361)
  line L86 (23.5063, 31.361) -> (24.3309, 31.361)
  spline S22 degree 2 poles (24.3309, 31.361) (24.6058, 31.361) (24.9767, 31.3013) (25.1452, 31.1924) knots 0 0 0 1 2 2 2
  spline S23 degree 2 poles (25.1452, 31.1924) (25.3138, 31.0835) (25.5083, 30.7438) (25.5083, 30.4923) knots 0 0 0 1 2 2 2
  spline S24 degree 2 poles (25.5083, 30.4923) (25.5083, 30.1422) (25.1504, 29.6676) (24.8444, 29.5535) knots 0 0 0 1 2 2 2
  line L87 (24.8444, 29.5535) -> (25.9828, 28.161)
  spline S25 degree 2 poles (25.0648, 30.4586) (25.0648, 30.5986) (24.9663, 30.8138) (24.8626, 30.8838) knots 0 0 0 1 2 2 2
  spline S26 degree 2 poles (24.8626, 30.8838) (24.7718, 30.9435) (24.5306, 30.9927) (24.3543, 30.9927) knots 0 0 0 1 2 2 2
  line L88 (24.3543, 30.9927) -> (23.9316, 30.9927)
  line L89 (23.9316, 30.9927) -> (23.9316, 29.7895)
  line L90 (23.9316, 29.7895) -> (24.305, 29.7895)
  spline S27 degree 2 poles (24.305, 29.7895) (24.4891, 29.7895) (24.7822, 29.8543) (24.8833, 29.9555) knots 0 0 0 1 2 2 2
  spline S28 degree 2 poles (24.8833, 29.9555) (24.9767, 30.0436) (25.0648, 30.2926) (25.0648, 30.4586) knots 0 0 0 1 2 2 2
  spline S29 degree 2 poles (27.5776, 28.0987) (27.2379, 28.0987) (26.6752, 28.3062) (26.4729, 28.5162) knots 0 0 0 1 2 2 2
  spline S30 degree 2 poles (26.4729, 28.5162) (26.2707, 28.7289) (26.0554, 29.3564) (26.0554, 29.7636) knots 0 0 0 1 2 2 2
  spline S31 degree 2 poles (26.0554, 29.7636) (26.0554, 30.15) (26.2732, 30.762) (26.4755, 30.9798) knots 0 0 0 1 2 2 2
  spline S32 degree 2 poles (26.4755, 30.9798) (26.67, 31.1898) (27.2405, 31.418) (27.5802, 31.418) knots 0 0 0 1 2 2 2
  spline S33 degree 2 poles (27.5802, 31.418) (27.7436, 31.418) (28.0392, 31.3714) (28.1741, 31.3299) knots 0 0 0 1 2 2 2
  spline S34 degree 2 poles (28.1741, 31.3299) (28.283, 31.2987) (28.5475, 31.1846) (28.6279, 31.1432) knots 0 0 0 1 2 2 2
  line L91 (28.6279, 31.1432) -> (28.6279, 30.6297)
  line L92 (28.6279, 30.6297) -> (28.5916, 30.6297)
  spline S35 degree 2 poles (28.5916, 30.6297) (28.5112, 30.6997) (28.3426, 30.8268) (28.187, 30.8994) knots 0 0 0 1 2 2 2
  spline S36 degree 2 poles (28.187, 30.8994) (28.0574, 30.9642) (27.7228, 31.0498) (27.5309, 31.0498) knots 0 0 0 1 2 2 2
  spline S37 degree 2 poles (27.5309, 31.0498) (27.0694, 31.0498) (26.4989, 30.3548) (26.4989, 29.7765) knots 0 0 0 1 2 2 2
  spline S38 degree 2 poles (26.4989, 29.7765) (26.4989, 29.455) (26.6493, 28.9727) (26.7919, 28.8067) knots 0 0 0 1 2 2 2
  spline S39 degree 2 poles (26.7919, 28.8067) (26.9293, 28.6407) (27.3183, 28.467) (27.5621, 28.467) knots 0 0 0 1 2 2 2
  spline S40 degree 2 poles (27.5621, 28.467) (27.741, 28.467) (28.0989, 28.5188) (28.2207, 28.5707) knots 0 0 0 1 2 2 2
  line L93 (28.2207, 28.5707) -> (28.2207, 29.3979)
  line L94 (28.2207, 29.3979) -> (27.4791, 29.3979)
  line L95 (27.4791, 29.3979) -> (27.4791, 29.7714)
  line L96 (27.4791, 29.7714) -> (28.6408, 29.7714)
  line L97 (28.6408, 29.7714) -> (28.6408, 28.3736)
  spline S41 degree 2 poles (28.6408, 28.3736) (28.5604, 28.3373) (28.2856, 28.2258) (28.1689, 28.1921) knots 0 0 0 1 2 2 2
  spline S42 degree 2 poles (28.1689, 28.1921) (28.0107, 28.1454) (27.7566, 28.0987) (27.5776, 28.0987) knots 0 0 0 1 2 2 2
  line L98 (29.175, 28.161) -> (29.175, 31.361)
  line L99 (29.175, 31.361) -> (31.177, 31.361)
  line L100 (31.177, 31.361) -> (31.177, 30.9824)
  line L101 (31.177, 30.9824) -> (29.6003, 30.9824)
  line L102 (29.6003, 30.9824) -> (29.6003, 30.1059)
  line L103 (29.6003, 30.1059) -> (31.0707, 30.1059)
  line L104 (31.0707, 30.1059) -> (31.0707, 29.7273)
  line L105 (31.0707, 29.7273) -> (29.6003, 29.7273)
  line L106 (29.6003, 29.7273) -> (29.6003, 28.5396)
  line L107 (29.6003, 28.5396) -> (31.177, 28.5396)
  line L108 (31.177, 28.5396) -> (31.177, 28.161)
  line L109 (31.177, 28.161) -> (29.175, 28.161)
  spline S43 degree 2 poles (32.5358, 28.1039) (32.1883, 28.1039) (31.7008, 28.2492) (31.4856, 28.3529) knots 0 0 0 1 2 2 2
  line L110 (31.4856, 28.3529) -> (31.4856, 28.8871)
  line L111 (31.4856, 28.8871) -> (31.5167, 28.8871)
  spline S44 degree 2 poles (31.5167, 28.8871) (31.7267, 28.69) (32.2583, 28.4722) (32.5047, 28.4722) knots 0 0 0 1 2 2 2
  spline S45 degree 2 poles (32.5047, 28.4722) (32.8574, 28.4722) (33.2178, 28.7652) (33.2178, 29.0064) knots 0 0 0 1 2 2 2
  spline S46 degree 2 poles (33.2178, 29.0064) (33.2178, 29.1983) (33.0285, 29.4368) (32.8237, 29.4965) knots 0 0 0 1 2 2 2
  spline S47 degree 2 poles (32.8237, 29.4965) (32.6758, 29.538) (32.4295, 29.595) (32.2454, 29.6417) knots 0 0 0 1 2 2 2
  spline S48 degree 2 poles (32.2454, 29.6417) (32.0794, 29.6858) (31.8175, 29.818) (31.7164, 29.9244) knots 0 0 0 1 2 2 2
  spline S49 degree 2 poles (31.7164, 29.9244) (31.6178, 30.0307) (31.5089, 30.3159) (31.5089, 30.5026) knots 0 0 0 1 2 2 2
  spline S50 degree 2 poles (31.5089, 30.5026) (31.5089, 30.8916) (32.1157, 31.418) (32.5851, 31.418) knots 0 0 0 1 2 2 2
  spline S51 degree 2 poles (32.5851, 31.418) (32.8548, 31.418) (33.3319, 31.3117) (33.5368, 31.2106) knots 0 0 0 1 2 2 2
  line L112 (33.5368, 31.2106) -> (33.5368, 30.7023)
  line L113 (33.5368, 30.7023) -> (33.5057, 30.7023)
  spline S52 degree 2 poles (33.5057, 30.7023) (33.3527, 30.8423) (32.8755, 31.0498) (32.6136, 31.0498) knots 0 0 0 1 2 2 2
  spline S53 degree 2 poles (32.6136, 31.0498) (32.318, 31.0498) (31.9523, 30.7723) (31.9523, 30.5467) knots 0 0 0 1 2 2 2
  spline S54 degree 2 poles (31.9523, 30.5467) (31.9523, 30.3445) (32.1676, 30.1033) (32.3698, 30.0488) knots 0 0 0 1 2 2 2
  spline S55 degree 2 poles (32.3698, 30.0488) (32.5047, 30.0125) (32.8963, 29.9192) (33.0259, 29.8803) knots 0 0 0 1 2 2 2
  spline S56 degree 2 poles (33.0259, 29.8803) (33.3553, 29.7791) (33.6613, 29.372) (33.6613, 29.0738) knots 0 0 0 1 2 2 2
  spline S57 degree 2 poles (33.6613, 29.0738) (33.6613, 28.8845) (33.5083, 28.5214) (33.3708, 28.3944) knots 0 0 0 1 2 2 2
  spline S58 degree 2 poles (33.3708, 28.3944) (33.2178, 28.2543) (32.8288, 28.1039) (32.5358, 28.1039) knots 0 0 0 1 2 2 2
  spline S59 degree 2 poles (43.1368, 29.1438) (43.1368, 28.9052) (42.9553, 28.5396) (42.8049, 28.4203) knots 0 0 0 1 2 2 2
  spline S60 degree 2 poles (42.8049, 28.4203) (42.6233, 28.2803) (42.211, 28.161) (41.8843, 28.161) knots 0 0 0 1 2 2 2
  line L114 (41.8843, 28.161) -> (40.9663, 28.161)
  line L115 (40.9663, 28.161) -> (40.9663, 31.361)
  line L116 (40.9663, 31.361) -> (41.8143, 31.361)
  spline S61 degree 2 poles (41.8143, 31.361) (42.1566, 31.361) (42.4989, 31.3169) (42.6544, 31.2313) knots 0 0 0 1 2 2 2
  spline S62 degree 2 poles (42.6544, 31.2313) (42.8282, 31.1406) (42.9864, 30.8423) (42.9864, 30.6401) knots 0 0 0 1 2 2 2
  spline S63 degree 2 poles (42.9864, 30.6401) (42.9864, 30.4145) (42.7478, 30.0566) (42.5378, 29.9555) knots 0 0 0 1 2 2 2
  line L117 (42.5378, 29.9555) -> (42.5378, 29.9399)
  spline S64 degree 2 poles (42.5378, 29.9399) (42.823, 29.8621) (43.1368, 29.4498) (43.1368, 29.1438) knots 0 0 0 1 2 2 2
  spline S65 degree 2 poles (42.6933, 29.1256) (42.6933, 29.3072) (42.5896, 29.5406) (42.434, 29.6235) knots 0 0 0 1 2 2 2
  spline S66 degree 2 poles (42.434, 29.6235) (42.3329, 29.6754) (42.0943, 29.7065) (41.8739, 29.7065) knots 0 0 0 1 2 2 2
  line L118 (41.8739, 29.7065) -> (41.3916, 29.7065)
  line L119 (41.3916, 29.7065) -> (41.3916, 28.524)
  line L120 (41.3916, 28.524) -> (41.7365, 28.524)
  spline S67 degree 2 poles (41.7365, 28.524) (42.0165, 28.524) (42.3381, 28.5759) (42.4626, 28.6589) knots 0 0 0 1 2 2 2
  spline S68 degree 2 poles (42.4626, 28.6589) (42.5818, 28.7445) (42.6933, 28.9571) (42.6933, 29.1256) knots 0 0 0 1 2 2 2
  spline S69 degree 2 poles (42.5429, 30.5804) (42.5429, 30.6945) (42.4651, 30.8657) (42.3796, 30.915) knots 0 0 0 1 2 2 2
  spline S70 degree 2 poles (42.3796, 30.915) (42.2758, 30.972) (42.0243, 30.9979) (41.7987, 30.9979) knots 0 0 0 1 2 2 2
  line L121 (41.7987, 30.9979) -> (41.3916, 30.9979)
  line L122 (41.3916, 30.9979) -> (41.3916, 30.0618)
  line L123 (41.3916, 30.0618) -> (41.8739, 30.0618)
  spline S71 degree 2 poles (41.8739, 30.0618) (42.0736, 30.0618) (42.2629, 30.1033) (42.364, 30.1681) knots 0 0 0 1 2 2 2
  spline S72 degree 2 poles (42.364, 30.1681) (42.4626, 30.2303) (42.5429, 30.43) (42.5429, 30.5804) knots 0 0 0 1 2 2 2
  spline S73 degree 2 poles (47.1044, 29.1438) (47.1044, 28.9052) (46.9228, 28.5396) (46.7724, 28.4203) knots 0 0 0 1 2 2 2
  spline S74 degree 2 poles (46.7724, 28.4203) (46.5909, 28.2803) (46.1786, 28.161) (45.8519, 28.161) knots 0 0 0 1 2 2 2
  line L124 (45.8519, 28.161) -> (44.9339, 28.161)
  line L125 (44.9339, 28.161) -> (44.9339, 31.361)
  line L126 (44.9339, 31.361) -> (45.7818, 31.361)
  spline S75 degree 2 poles (45.7818, 31.361) (46.1241, 31.361) (46.4664, 31.3169) (46.622, 31.2313) knots 0 0 0 1 2 2 2
  spline S76 degree 2 poles (46.622, 31.2313) (46.7958, 31.1406) (46.954, 30.8423) (46.954, 30.6401) knots 0 0 0 1 2 2 2
  spline S77 degree 2 poles (46.954, 30.6401) (46.954, 30.4145) (46.7154, 30.0566) (46.5053, 29.9555) knots 0 0 0 1 2 2 2
  line L127 (46.5053, 29.9555) -> (46.5053, 29.9399)
  spline S78 degree 2 poles (46.5053, 29.9399) (46.7906, 29.8621) (47.1044, 29.4498) (47.1044, 29.1438) knots 0 0 0 1 2 2 2
  spline S79 degree 2 poles (46.6609, 29.1256) (46.6609, 29.3072) (46.5572, 29.5406) (46.4016, 29.6235) knots 0 0 0 1 2 2 2
  spline S80 degree 2 poles (46.4016, 29.6235) (46.3005, 29.6754) (46.0619, 29.7065) (45.8415, 29.7065) knots 0 0 0 1 2 2 2
  line L128 (45.8415, 29.7065) -> (45.3591, 29.7065)
  line L129 (45.3591, 29.7065) -> (45.3591, 28.524)
  line L130 (45.3591, 28.524) -> (45.704, 28.524)
  spline S81 degree 2 poles (45.704, 28.524) (45.9841, 28.524) (46.3057, 28.5759) (46.4301, 28.6589) knots 0 0 0 1 2 2 2
  spline S82 degree 2 poles (46.4301, 28.6589) (46.5494, 28.7445) (46.6609, 28.9571) (46.6609, 29.1256) knots 0 0 0 1 2 2 2
  spline S83 degree 2 poles (46.5105, 30.5804) (46.5105, 30.6945) (46.4327, 30.8657) (46.3472, 30.915) knots 0 0 0 1 2 2 2
  spline S84 degree 2 poles (46.3472, 30.915) (46.2434, 30.972) (45.9919, 30.9979) (45.7663, 30.9979) knots 0 0 0 1 2 2 2
  line L131 (45.7663, 30.9979) -> (45.3591, 30.9979)
  line L132 (45.3591, 30.9979) -> (45.3591, 30.0618)
  line L133 (45.3591, 30.0618) -> (45.8415, 30.0618)
  spline S85 degree 2 poles (45.8415, 30.0618) (46.0412, 30.0618) (46.2305, 30.1033) (46.3316, 30.1681) knots 0 0 0 1 2 2 2
  spline S86 degree 2 poles (46.3316, 30.1681) (46.4301, 30.2303) (46.5105, 30.43) (46.5105, 30.5804) knots 0 0 0 1 2 2 2
  spline S87 degree 2 poles (50.1514, 28.1039) (49.8402, 28.1039) (49.3138, 28.314) (49.1219, 28.524) knots 0 0 0 1 2 2 2
  spline S88 degree 2 poles (49.1219, 28.524) (48.93, 28.7315) (48.7199, 29.3539) (48.7199, 29.7584) knots 0 0 0 1 2 2 2
  spline S89 degree 2 poles (48.7199, 29.7584) (48.7199, 30.1603) (48.9248, 30.7568) (49.1193, 30.9772) knots 0 0 0 1 2 2 2
  spline S90 degree 2 poles (49.1193, 30.9772) (49.3112, 31.1924) (49.835, 31.418) (50.1591, 31.418) knots 0 0 0 1 2 2 2
  spline S91 degree 2 poles (50.1591, 31.418) (50.3199, 31.418) (50.6026, 31.3714) (50.7219, 31.3351) knots 0 0 0 1 2 2 2
  spline S92 degree 2 poles (50.7219, 31.3351) (50.8256, 31.3013) (51.0408, 31.2054) (51.1472, 31.1483) knots 0 0 0 1 2 2 2
  line L134 (51.1472, 31.1483) -> (51.1472, 30.6349)
  line L135 (51.1472, 30.6349) -> (51.1134, 30.6349)
  spline S93 degree 2 poles (51.1134, 30.6349) (51.0564, 30.6868) (50.8801, 30.832) (50.753, 30.902) knots 0 0 0 1 2 2 2
  spline S94 degree 2 poles (50.753, 30.902) (50.6311, 30.9694) (50.3433, 31.055) (50.1566, 31.055) knots 0 0 0 1 2 2 2
  spline S95 degree 2 poles (50.1566, 31.055) (49.9517, 31.055) (49.5861, 30.8864) (49.4486, 30.7256) knots 0 0 0 1 2 2 2
  spline S96 degree 2 poles (49.4486, 30.7256) (49.3138, 30.5623) (49.1634, 30.067) (49.1634, 29.7584) knots 0 0 0 1 2 2 2
  spline S97 degree 2 poles (49.1634, 29.7584) (49.1634, 29.4291) (49.3215, 28.9545) (49.459, 28.7911) knots 0 0 0 1 2 2 2
  spline S98 degree 2 poles (49.459, 28.7911) (49.5938, 28.6329) (49.9543, 28.4722) (50.1566, 28.4722) knots 0 0 0 1 2 2 2
  spline S99 degree 2 poles (50.1566, 28.4722) (50.3407, 28.4722) (50.6544, 28.5629) (50.7763, 28.6303) knots 0 0 0 1 2 2 2
  spline S100 degree 2 poles (50.7763, 28.6303) (50.893, 28.6978) (51.0668, 28.8378) (51.116, 28.8871) knots 0 0 0 1 2 2 2
  line L136 (51.116, 28.8871) -> (51.1472, 28.8871)
  line L137 (51.1472, 28.8871) -> (51.1472, 28.3788)
  spline S101 degree 2 poles (51.1472, 28.3788) (51.0408, 28.3295) (50.8541, 28.2388) (50.7219, 28.1973) knots 0 0 0 1 2 2 2
  spline S102 degree 2 poles (50.7219, 28.1973) (50.5818, 28.1506) (50.3433, 28.1039) (50.1514, 28.1039) knots 0 0 0 1 2 2 2
  point P0 (28.8675, 0)
  dimension "d177" = 9.4743
  dimension "d178" = 4.8327
  constraints: 6 end point, 6 point on line, 2 perpendicular, 1 parallel, 2 other
  measures "d177" distance of L5.start L5.end
  measures "d178" distance of L7.start L7.end
extrude "Extrusion17" cut sketch "Sketch17" against normal blind 1.5 contours S76 S77 L4 | L4 S77 L127 S78 S74 L124 L125 L126 S75 S76 | S78 S73 S74 L4 | L9 L10 L11 L12 L13 L14 L15 L16 L17 L18 L19 L20 L21 | L22 L23 L24 L25 L26 L27 L28 L29 | S0 S1 L33 L34 L35 L36 L37 S2 S3 | L41 L42 L43 L44 L45 L46 | L47 L48 L49 L50 L51 L52 L53 L54 L55 L56 L57 L58 | S8 S9 L59 L60 L61 S10 S11 S12 L62 S13 | L69 L70 L71 L72 L73 L74 L75 L76 | L80 L81 L82 L83 L84 L85 L86 S22 S23 S24 L87 | S29 S30 S31 S32 S33 S34 L91 L92 S35 S36 S37 S38 S39 S40 L93 L94 L95 L96 L97 S41 S42 | L98 L99 L100 L101 L102 L103 L104 L105 L106 L107 L108 L109 | S43 L110 L111 S44 S45 S46 S47 S48 S49 S50 S51 L112 L113 S52 S53 S54 S55 S56 S57 S58 | S59 S60 L114 L115 L116 S61 S62 S63 L117 S64 | S87 S88 S89 S90 S91 S92 L134 L135 S93 S94 S95 S96 S97 S98 S99 S100 L136 L137 S101 S102